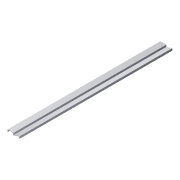
# Autodesk Inventor part: Wireholder
Saved by Autodesk Inventor 2016 (Build 200138000, 138)
## iProperties
Created: 2015-05-19
Part Number: Wireholder
Material: Aluminum 6061
Document SubType Name: Modeling
Designer: Andy
Density: 2.7 g/cm^3
Appearance: Aluminum - Flat
Mass: 153.688 g
Surface Area: 1173.84 cm^2
Volume: 56.9214 cm^3
Author: Andy
Autodesk Inventor part; units mm, degrees
ref_plane "YZ Plane" through (0, 0, 0) normal (1, 0, 0) x (0, 1, 0)
ref_plane "XZ Plane" through (0, 0, 0) normal (0, 1, 0) x (-1, 0, 0)
ref_plane "XY Plane" through (0, 0, 0) normal (0, 0, 1) x (1, 0, 0)
sketch "Sketch1" plane through (0, 0, 0) normal (0, 1, 0) x (-1, 0, 0)
  line L0 (0, 0) -> (56, 0)
  line L1 (56, 0) -> (56, -10)
  line L2 (56, -10) -> (0, -10)
  line L3 (0, -10) -> (0, 0)
  line L4 (55, -10) -> (55, -1)
  line L5 (55, -1) -> (29, -1)
  line L6 (29, -1) -> (29, -10)
  line L7 (29, -10) -> (55, -10)
  line L8 (1, -10) -> (1, -1)
  line L9 (29, -10) -> (28, -10)
  line L10 (28, -10) -> (1, -1)
  line L11 (28, 0) -> (28, -9)
  line L12 (28, -9) -> (1, 0)
  dimension "d0" = 56
  dimension "d1" = 10
  dimension "d2" = 9
  dimension "d3" = 26
  dimension "d4" = 9
  constraints: 26 end point, 6 perpendicular, 3 point on line, 2 midpoint, 2 parallel, 1 horizontal, 1 vertical
  measures "d0" distance of L0.start L0.end
  measures "d1" distance of L0.end L1.end
  measures "d2" distance of L4.start L4.end
  measures "d3" distance of L5.end L4.end
  measures "d4" distance of L11.start L11.end
extrude "Extrusion1" add sketch "Sketch1" along normal blind 711.2 contours L0 L12 L11 L1 L2 L4 L5 L6 L10 L8 L3
body "Solid1"
